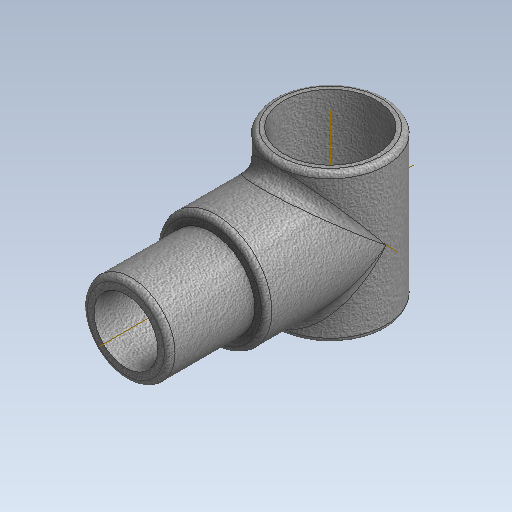
# Autodesk Inventor part: L114-6
Saved by Autodesk Inventor 2021 (Build 250183000, 183)
## iProperties
Created: 2020-04-23
Part Number: L114-6
Material: Aluminium Cast
Document SubType Name: Modeling
Designer: Hannah
Density: 2.9519 g/cm^3
Appearance: Aluminum Cast
Mass: 180 g
Surface Area: 246.767 cm^2
Volume: 60.9777 cm^3
Vendor: Kee Systems
Description: swivel tee
Catalog Web Link: https://keesystems.com/store/fittings/kee-lite/l114-swivel-tee.html
Size: 6
Length: n/a
OD: n/a
Author: Hannah
Revision Number: -
Autodesk Inventor part; units mm, degrees
ref_plane "YZ Plane" through (0, 0, 0) normal (1, 0, 0) x (0, 1, 0)
ref_plane "XZ Plane" through (0, 0, 0) normal (0, 1, 0) x (-1, 0, 0)
ref_plane "XY Plane" through (0, 0, 0) normal (0, 0, 1) x (1, 0, 0)
sketch "Sketch1" plane through (0, 0, 0) normal (0, 0, 1) x (1, 0, 0)
  circle A0 centre (0, 0) radius 16.5
  circle A1 centre (0, 0) radius 21
  circle A2 centre (0, 0) radius 12
  dimension "d1" = 42
  dimension "d2" = 33
  dimension "d34" = 24
  constraints: 3 centre point, 3 coincident
  measures "d1" diameter of A1
  measures "d2" diameter of A0
  measures "d34" diameter of A2
extrude "Extrusion1" add sketch "Sketch1" along normal blind 45 contours A0 | A1 | A2
sketch "Sketch2" plane through (0, 0, 0) normal (0, 1, 0) x (-1, 0, 0)
  circle A0 centre (0, 0) radius 17.5
  circle A1 centre (0, 0) radius 21
  dimension "d5" = 35
  dimension "d6" = 42
  constraints: 2 centre point, 2 coincident
  measures "d5" diameter of A0
  measures "d6" diameter of A1
extrude "Extrusion2" add sketch "Sketch2" along normal mid plane 56 contours A0 | A1
extrude "Extrusion4" add sketch "Sketch1" along normal blind 32 from surface at 45 contours A0 | A2
extrude "Extrusion3" cut sketch "Sketch2" against normal up to surface (56 mm away) from surface at 28 contours A0
extrude "Extrusion5" cut sketch "Sketch1" along normal through all contours A2
fillet "Fillet1" radius 5 2 edges at (0, 21, 21) (0, -21, 21)
hole "Hole1" at (0, 0, 0) direction (-1, 0, 0) diameter 8.376 end through all thread size "M10x1.5" class "6H" standard "ISO Metric profile"
fillet "Fillet2" radius 2 4 edges at (21, 28, 0) (21, -28, 0) (-16.5, 0, 77) (-21, 0, 45)
equation "\"d34\" = 2 * d2 - d1"
equation "\"d6\" = d1"
body "Solid1"
